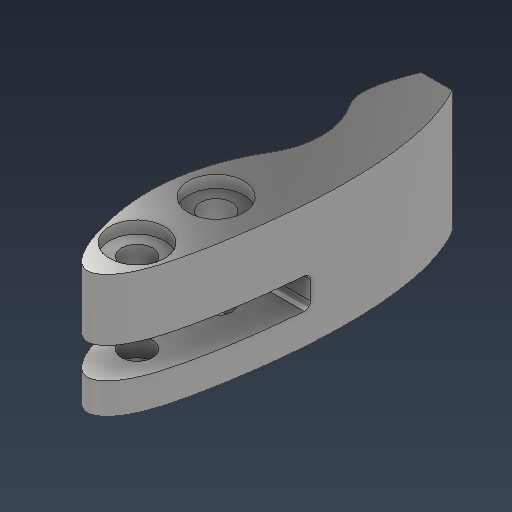
# Autodesk Inventor part: holder3_l2
Saved by Autodesk Inventor 2021 (Build 250183000, 183)
## iProperties
Created: 2021-06-13
Part Number: holder3_l2
Material: Steel, Mild
Document SubType Name: Modeling
Designer: Watchdog
Density: 7.85 g/cm^3
Appearance: Semi-Polished
Mass: 69.0338 g
Surface Area: 42.8037 cm^2
Volume: 8.79411 cm^3
Author: Watchdog
Autodesk Inventor part; units mm, degrees
ref_plane "XZ Plane" through (0, 0, 0) normal (0, 1, 0) x (-1, 0, 0)
ref_plane "XY Plane" through (0, 0, 0) normal (0, 0, 1) x (1, 0, 0)
sketch "Sketch1" plane through (0, 0, 0) normal (0, 1, 0) x (-1, 0, 0)
  line L0 (-12.113, 0) -> (-12.113, -47.112)
  arc A0 (-10.113, -23.3328) -> (-10.113, -36.6672) centre (0, -30) ccw
  spline S0 degree 2 poles (-10.113, -36.6672) (-8.0323, -39.3688) (-11.3054, -47.112) knots 0 0 0 1 1 1
  line L1 (-11.3054, -47.112) -> (-16.3054, -47.112)
  line L2 (-16.3054, -47.112) -> (-22.824, -35.4482) construction
  line L3 (-22.824, -35.4482) -> (-19.0316, -2.7043) construction
  line L4 (-19.0316, -2.7043) -> (-16.3054, 5.9052) construction
  line L5 (-16.3054, 5.9052) -> (-10.5542, 11.5518) construction
  line L6 (-10.5542, 11.5518) -> (-6.122, 0.697) construction
  line L7 (-6.122, 0.697) -> (-4.6066, -13.5917) construction
  line L8 (-4.6066, -13.5917) -> (-10.113, -23.3328) construction
  spline S1 degree 4 poles (-16.3054, -47.112) (-22.824, -35.4482) (-19.0316, -2.7043) (-16.3054, 5.9052) (-10.5542, 11.5518) (-6.122, 0.697) (-4.6066, -13.5917) (-10.113, -23.3328) knots 0 0 0 0 0 1 2 3 4 4 4 4 4
  point P0 (0, 0)
  point P1 (-12.113, -30)
  point P2 (-12.113, -12.887)
  point P3 (-9.3056, -39.3909)
  dimension "d0" = 47.112
  dimension "d1" = 0
  dimension "d2" = 12.113
  dimension "d3" = 30
  dimension "d4" = 12.887
  dimension "d5" = 12.113
  dimension "d6" = 2
  dimension "d7" = 2
  dimension "d8" = 5
  constraints: 4 end point, 3 point on circle, 2 point on line, 1 centre point, 1 horizontal, 1 tangent, 1 vertical, 6 other
  measures "d0" distance of L0.start L0.end
  measures "d1" vertical distance of point (0, 0) L0.start
  measures "d2" distance of point (0, 0) L0.start
  measures "d3" distance of L0.start point (-12.113, -30)
  measures "d4" distance of L0.start point (-12.113, -12.887)
  measures "d5" radius of A0
  measures "d6" horizontal distance of L0.end A0.end
  measures "d7" horizontal distance of L0.end L8.end
  measures "d8" distance of L1.start L1.end
extrude "Extrusion1" add sketch "Sketch1" along normal blind 20
sketch "Sketch2" plane through (0, 20, 0) normal (0, 1, 0) x (1, 0, 0)
  point P0 (0, 0)
  point P1 (12.133, 0)
  point P2 (12.133, 12.877)
  dimension "d11" = 12.133
  dimension "d12" = 0
  dimension "d13" = 12.877
  measures "d11" distance of point (0, 0) point (12.133, 0)
  measures "d12" horizontal distance of point (12.133, 12.877) point (12.133, 0)
  measures "d13" distance of point (12.133, 0) point (12.133, 12.877)
hole "Hole1" at (12.133, 20, 0) at (12.133, 20, -12.877) direction (0, -1, 0) diameter 5 end through all
ref_plane "Work Plane1" through (5.8904, 10, -8.1838) normal (-1, 0, 0) x (0, -1, 0)
sketch "Sketch3" plane through (5.8904, 10, -8.1838) normal (-1, 0, 0) x (0, -1, 0)
  line L0 (0, -11.6932) -> (5, -11.6932)
  line L1 (5, -11.6932) -> (5, 38.3068)
  line L2 (5, 38.3068) -> (0, 38.3068)
  line L3 (0, 38.3068) -> (0, -11.6932)
  line L4 (10, 10.6838) -> (10, 5.6838) projected
  line L5 (-10, 5.6838) -> (-10, 10.6838) projected
  line L6 (10, -2.1932) -> (10, -7.1932) projected
  line L7 (-10, -7.1932) -> (-10, -2.1932) projected
  point P0 (10, 8.1838)
  dimension "d22" = 5
  dimension "d23" = 20
  dimension "d24" = 10
  dimension "d25" = 50
  dimension "d29" = 5
  dimension "d30" = 4.5
  constraints: 8 end point, 2 parallel, 1 horizontal, 1 perpendicular
  measures "d22" distance between parallel lines of L1 L3
  measures "d23" distance between parallel lines of L4 L5
  measures "d24" distance between parallel lines of L3 L5
  measures "d25" distance between parallel lines of L0 L2
  measures "d29" distance of L7.start L7.end
  measures "d30" distance from line of L0 L7.start
extrude "Extrusion2" cut sketch "Sketch3" against normal through all
fillet "Fillet1" radius 1 2 edges at (14.4446, 10, -19.877) (14.4446, 5, -19.877)
sketch "Sketch4" plane through (0, 20, 0) normal (0, 1, 0) x (1, 0, 0)
  circle A0 centre (12.133, 12.877) radius 2.5 projected
  circle A1 centre (12.133, 0) radius 2.5 projected
  circle A2 centre (12.133, 12.877) radius 4.5
  circle A3 centre (12.133, 0) radius 4.5
  point P0 (0, 0)
  dimension "d31" = 2
  dimension "d32" = 2
  constraints: 2 centre point
  measures "d31" radial gap between concentric circles of A0 A2
  measures "d32" radial gap between concentric circles of A1 A3
extrude "Extrusion3" cut sketch "Sketch4" against normal blind 2
sketch "Sketch5" plane through (0, 0, 0) normal (0, -1, 0) x (1, 0, 0)
  circle A0 centre (12.133, -12.877) radius 2.5 projected
  circle A1 centre (12.133, 0) radius 2.5 projected
  circle A2 centre (12.133, -12.877) radius 4.5
  circle A3 centre (12.133, 0) radius 4.5
  point P0 (0, 0)
  dimension "d35" = 2
  dimension "d36" = 2
  constraints: 2 centre point
  measures "d35" radial gap between concentric circles of A0 A2
  measures "d36" radial gap between concentric circles of A1 A3
extrude "Extrusion4" cut sketch "Sketch5" against normal blind 2
equation "\"d5\" = d2"
equation "\"d7\" = d6"
body "Solid1"
